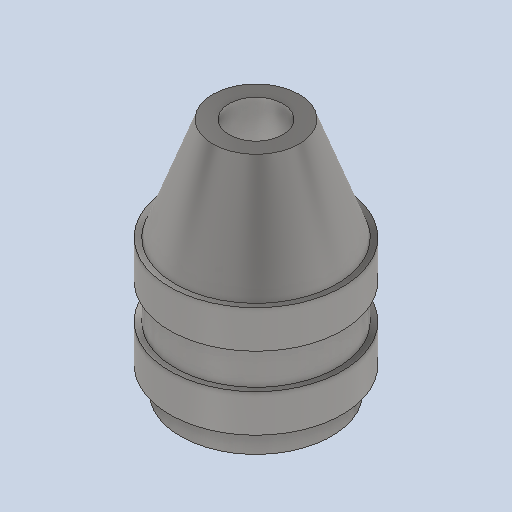
# Autodesk Inventor part: B3OFT4_HF2_kezifuro_Tokmany
Saved by Autodesk Inventor 2023.3 (Build 273359000, 359)
## iProperties
Created: 2023-11-30
Part Number: B3OFT4_HF2_kezifuro_Tokmany
Material: Stainless Steel
Document SubType Name: Modeling
Designer: Csábi-Kis Henrik
Density: 8 g/cm^3
Appearance: Semi-Polished
Mass: 150.457 g
Surface Area: 74.0907 cm^2
Volume: 18.8071 cm^3
Author: Csábi-Kis Henrik
Autodesk Inventor part; units mm, degrees
ref_plane "YZ Plane" through (0, 0, 0) normal (1, 0, 0) x (0, 1, 0)
ref_plane "XZ Plane" through (0, 0, 0) normal (0, 1, 0) x (-1, 0, 0)
ref_plane "XY Plane" through (0, 0, 0) normal (0, 0, 1) x (1, 0, 0)
sketch "Sketch1" plane through (0, 0, 0) normal (0, 0, 1) x (1, 0, 0)
  line L0 (0, 52.8) -> (0, -8.8) construction
  line L1 (-18, 0) -> (3, 0) construction
  line L2 (-15, 0) -> (0, 0)
  line L3 (-15, 0) -> (-15, 25)
  line L4 (-15, 25) -> (-8, 44)
  line L5 (-8, 44) -> (0, 44)
  line L6 (0, 44) -> (0, 0)
  line L7 (-15, 0) -> (-14, 0)
  line L8 (-14, 0) -> (-14, 4.5)
  line L9 (-14, 4.5) -> (-15, 4.5)
  line L10 (-15, 4.5) -> (-15, 0)
  dimension "d0" = 15
  dimension "d1" = 44
  dimension "d2" = 8
  dimension "d3" = 25
  dimension "d31" = 1
  dimension "d32" = 4.5
  constraints: 18 end point, 3 perpendicular, 2 parallel, 2 point on line, 1 collinear, 1 horizontal, 1 vertical
  measures "d0" distance of L2.end L2.start
  measures "d1" distance between parallel lines of L1 L5
  measures "d2" distance of L4.end L5.end
  measures "d3" distance of L2.start L3.end
  measures "d31" distance of L8.end L9.end
  measures "d32" distance of L7.end L8.end
revolve "Revolution1" add sketch "Sketch1" angle 360 about axis through (0, 0, 0) along (0, -1, 0)
revolve "Revolution4" cut sketch "Sketch1" angle 360 about axis through (0, 0, 0) along (0, -1, 0) contours L3 L9 L8 L2
sketch "Sketch2" plane through (0, 0, 0) normal (0, 0, 1) x (1, 0, 0)
  line L0 (-8, 44) -> (-15, 25) projected
  line L1 (-8, 44) -> (8, 44) projected
  line L2 (8, 44) -> (15, 25) projected
  line L3 (0, 44) -> (0, 20)
  line L4 (0, 20) -> (-12, 20)
  line L5 (-5, 44) -> (-12, 20)
  line L6 (0, 15.2) -> (0, 48.8) projected
  dimension "d10" = 12
  dimension "d11" = 3
  dimension "d12" = 24
  constraints: 6 end point, 1 midpoint, 1 perpendicular, 1 point on line, 1 vertical
  measures "d10" distance of L3.end L4.end
  measures "d11" distance of L0.start L5.start
  measures "d12" distance of L3.start L3.end
revolve "Revolution2" cut sketch "Sketch2" angle 360 about axis through (0, -10, 0) along (0, 1, 0)
sketch "Sketch3" plane through (0, 0, 0) normal (0, -1, 0) x (1, 0, 0)
  circle A0 centre (0, 0) radius 15 projected
hole "Hole1" at (0, 0, 0) direction (0, 1, 0) diameter 11.835 depth 20 thread size "M14x2" class "6H" standard "ISO Metric profile"
sketch "Sketch4" plane through (0, 0, 0) normal (0, 0, 1) x (1, 0, 0)
  line L0 (-15, 0) -> (15, 0) projected
  line L1 (-15, 25) -> (15, 25) projected
  line L2 (-15, 25) -> (-15, 0)
  line L3 (-15, 25) -> (-16, 25)
  line L4 (-16, 25) -> (-16, 18)
  line L5 (-16, 18) -> (-15, 18)
  line L6 (-15, 18) -> (-15, 25)
  line L7 (-15, 11.5) -> (-16, 11.5)
  line L8 (-16, 11.5) -> (-16, 4.5)
  line L9 (-16, 4.5) -> (-15, 4.5)
  line L10 (-15, 4.5) -> (-15, 11.5)
  line L11 (0, -5) -> (0, 30) projected
  line L12 (15, 4.5) -> (-15, 4.5) projected
  point P0 (-15.5, 11.5)
  point P1 (-15.5, 18)
  point P2 (-15, 8)
  point P3 (-15, 18)
  dimension "d24" = 1
  dimension "d28" = 7
  dimension "d29" = 7
  constraints: 18 end point, 5 parallel, 2 horizontal, 2 midpoint, 2 perpendicular, 1 point on line, 1 vertical
  measures "d24" distance of L1.start L3.end
  measures "d28" distance of L7.end L8.end
  measures "d29" distance of L3.end L4.end
revolve "Revolution3" add sketch "Sketch4" angle 360 about axis through (0, -10, 0) along (0, 1, 0) contours L9 L8 L7 L2 | L5 L4 L3 L2
body "Solid1"
